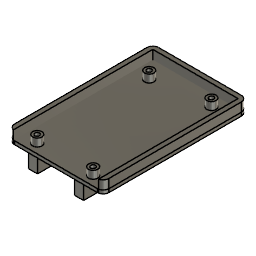
arduinoMount4080 (Autodesk Fusion 360 design; units mm, degrees)
part number: 2026-01-29-15-29-34-594
Autodesk Fusion 360 part; units mm, degrees
sketch "Sketch5" plane through (0, 0, 0) normal (0, 0, 1) x (1, 0, 0)
  line L0 (-41, -62.5) -> (41, -62.5)
  line L1 (41, -62.5) -> (41, 62.5)
  line L2 (41, 62.5) -> (-41, 62.5)
  line L3 (-41, 62.5) -> (-41, -62.5)
  line L4 (-41, -62.5) -> (41, 62.5) construction
  line L5 (41, -62.5) -> (-41, 62.5) construction
  line L6 (-37, 62.5) -> (-37, -62.5)
  line L7 (0, 62.5) -> (0, -62.5) construction
  line L8 (37, 62.5) -> (37, -62.5)
  line L9 (-10, -62.5) -> (10, -62.5) construction
  line L10 (23.95, -62.5) -> (16.05, -62.5)
  line L11 (16.05, -62.5) -> (16.05, 62.5)
  line L12 (16.05, 62.5) -> (23.95, 62.5)
  line L13 (23.95, 62.5) -> (23.95, -62.5)
  line L14 (-23.95, 62.5) -> (-23.95, -62.5)
  line L15 (-16.05, -62.5) -> (-16.05, 62.5)
  line L16 (-20, -62.5) -> (-20, 62.5) construction
  line L17 (20, -62.5) -> (20, 62.5) construction
  line L18 (-41, -58.5) -> (41, -58.5)
  line L19 (-23.95, -52.5) -> (-16.05, -52.5)
  line L20 (23.95, -52.5) -> (16.05, -52.5)
  line L21 (-27, -62.5) -> (-13, -62.5)
  line L22 (-13, -62.5) -> (-13, -72.5)
  line L23 (-13, -72.5) -> (-27, -72.5)
  line L24 (-27, -72.5) -> (-27, -62.5)
  line L25 (-27, -62.5) -> (-13, -72.5) construction
  line L26 (-27, -72.5) -> (-13, -62.5) construction
  circle A0 centre (-20, -67.5) radius 2.25
  line L27 (13, -72.5) -> (27, -72.5)
  line L28 (13, -62.5) -> (13, -72.5)
  line L29 (27, -72.5) -> (27, -62.5)
  circle A1 centre (20, -67.5) radius 2.25
  circle A2 centre (-24.25, -54.5) radius 4
  circle A3 centre (-24.25, -54.5) radius 2
  circle A4 centre (-23.75, 42.2) radius 4
  circle A5 centre (-23.75, 42.2) radius 2
  circle A6 centre (24.25, -54.5) radius 4
  circle A7 centre (24.25, -54.5) radius 2
  circle A8 centre (23.95, 48.5) radius 4
  circle A9 centre (23.95, 48.5) radius 2
  line L30 (-23.75, 42.2) -> (-23.75, 37.2315) construction
  line L31 (24.25, -54.5) -> (24.25, -58.0127) construction
  line L32 (-24.25, -54.5) -> (-24.25, -59.6718) construction
  line L33 (-41, 58.5) -> (41, 58.5)
  line L34 (-25.25, -56.2321) -> (-24.25, -56.8094)
  line L35 (-25.25, -56.2321) -> (-22.1514, -56.2321) construction
  line L36 (-23.25, -56.2321) -> (-24.25, -56.8094)
  line L37 (23.25, -56.2321) -> (24.25, -56.8094)
  line L38 (23.25, -56.2321) -> (25.465, -56.2321) construction
  line L39 (25.25, -56.2321) -> (24.25, -56.8094)
  line L40 (22.95, 46.7679) -> (23.95, 46.1906)
  line L41 (22.95, 46.7679) -> (25.5493, 46.7679) construction
  line L42 (24.95, 46.7679) -> (23.95, 46.1906)
  line L43 (-24.75, 40.4679) -> (-23.75, 39.8906)
  line L44 (-24.75, 40.4679) -> (-23.0984, 40.4679) construction
  line L45 (-22.75, 40.4679) -> (-23.75, 39.8906)
  dimension "d29" = 125
  dimension "d30" = 4
  dimension "d55" = 7.9
  dimension "d64" = 3.95
  dimension "d65" = 3.95
  dimension "d93" = 74
  dimension "d94" = 4
  dimension "d99" = 40
  dimension "d101" = 4
  dimension "d102" = 10
  dimension "d103" = 14
  dimension "d104" = 10
  dimension "d105" = 4.5
  dimension "d116" = 8
  dimension "d117" = 4
  dimension "d118" = 8
  dimension "d119" = 4
  dimension "d120" = 8
  dimension "d121" = 4
  dimension "d122" = 8
  dimension "d123" = 4
  dimension "d124" = 48.5
  dimension "d127" = 24.25
  dimension "d128" = 4
  dimension "d129" = 96.7
  dimension "d132" = 103
  dimension "d135" = 0.3
  dimension "d136" = 0.5
  dimension "d147" = 4
  dimension "d150" = 121
  dimension "d151" = 82
  dimension "d152" = 21
  dimension "d153" = 21
  dimension "d156" = 30
  dimension "d157" = 30
  dimension "d158" = 30
  dimension "d159" = 30
  constraint horizontal L0
  constraint perpendicular L0 L1
  constraint parallel L0 L2
  constraint parallel L1 L3
  constraint coincident L4 origin
  constraint coincident L5 origin
  constraint coincident L2 L6.start
  constraint coincident L0 L6.end
  constraint perpendicular L0 L6
  constraint midpoint L2 L7.start
  constraint midpoint L0 L7.end
  constraint symmetric L6.start L7 L8.start
  constraint symmetric L6.end L7 L8.end
  constraint horizontal L9
  constraint coincident L0 L9.start
  constraint horizontal L10
  constraint vertical L11
  constraint horizontal L12
  constraint vertical L13
  constraint coincident L0 L10.start
  constraint symmetric L7 L10.start L14.end
  constraint symmetric L7 L10.end L15.start
  constraint symmetric L7 L11.end L15.end
  constraint symmetric L7 L12.end L14.start
  constraint coincident L0 L16.start
  constraint coincident L2 L16.end
  constraint perpendicular L2 L16
  constraint symmetric L7 L16.start L17.start
  constraint symmetric L7 L16.end L17.end
  constraint coincident L2 L15.end
  constraint coincident L3 L18.start
  constraint coincident L1 L18.end
  constraint perpendicular L1 L18
  constraint coincident L14 L19.start
  constraint coincident L15 L19.end
  constraint perpendicular L15 L19
  constraint symmetric L7 L19.start L20.start
  constraint symmetric L7 L19.end L20.end
  constraint horizontal L21
  constraint vertical L22
  constraint horizontal L23
  constraint vertical L24
  constraint coincident L0 L21.start
  constraint midpoint L16.start L21
  constraint midpoint L25 A0.centre
  constraint symmetric L7 L21.start L29.end
  constraint symmetric L7 L21.end L28.start
  constraint symmetric L7 L22.end L27.start
  constraint symmetric L7 L23.end L27.end
  constraint symmetric L7 A0 A1
  constraint concentric A2 A3
  constraint concentric A4 A5
  constraint concentric A6 A7
  constraint concentric A8 A9
  constraint horizontal A2.centre A6.centre
  constraint vertical L30
  constraint coincident A4.centre A5.centre
  constraint vertical L31
  constraint coincident A6.centre A7.centre
  constraint vertical L32
  constraint coincident A2.centre A3.centre
  constraint coincident L3 L33.start
  constraint coincident L1 L33.end
  constraint perpendicular L1 L33
  constraint horizontal L35
  constraint coincident A3 L34.start
  constraint tangent A3 L34
  constraint coincident L32 L34.end
  constraint symmetric L32 L34.start L36.start
  constraint symmetric L32 L34.end L36.end
  constraint horizontal L38
  constraint coincident A7 L37.start
  constraint tangent A7 L37
  constraint coincident L31 L37.end
  constraint symmetric L31 L37.start L39.start
  constraint symmetric L31 L37.end L39.end
  constraint horizontal L41
  constraint coincident A9 L40.start
  constraint tangent A9 L40
  constraint coincident L13 L40.end
  constraint symmetric L13 L40.start L42.start
  constraint symmetric L13 L40.end L42.end
  constraint horizontal L44
  constraint coincident A5 L43.start
  constraint tangent A5 L43
  constraint coincident L30 L43.end
  constraint symmetric L30 L43.start L45.start
  constraint symmetric L30 L43.end L45.end
  measures "d29" distance of L0.end L1.end
  measures "d30" distance of L3 L6
  measures "d55" distance of L10.start L10.end
  measures "d64" distance of L14 L16
  measures "d65" distance of L15 L16
  measures "d93" distance of L6 L8
  measures "d94" distance of L1 L8
  measures "d99" distance of L16 L17
  measures "d101" distance of L0 L18
  measures "d102" distance of L16.start L19
  measures "d103" distance of L21.start L21.end
  measures "d104" distance of L21.start L23.end
  measures "d105" diameter of A0
  measures "d116" diameter of A2
  measures "d117" diameter of A3
  measures "d118" diameter of A4
  measures "d119" diameter of A5
  measures "d120" diameter of A6
  measures "d121" diameter of A7
  measures "d122" diameter of A8
  measures "d123" diameter of A9
  measures "d124" horizontal distance of A2.centre A6.centre
  measures "d127" distance of L7 A6.centre
  measures "d128" distance of L18 A6.centre
  measures "d129" vertical distance of A2.centre A4.centre
  measures "d132" vertical distance of A6.centre A8.centre
  measures "d135" horizontal distance of A6.centre A8.centre
  measures "d136" horizontal distance of A2.centre A4.centre
  measures "d147" distance of L2 L33
  measures "d150" distance of L0 L33
  measures "d151" distance of L1 L3
  measures "d152" distance of L3 L16
  measures "d153" distance of L1 L17
  measures "d156" angle of L34 L35
  measures "d157" angle of L37 L38
  measures "d158" angle of L40 L41
  measures "d159" angle of L43 L44
sketch "Sketch6" plane through (0, 0, 0) normal (0, 1, 0) x (1, 0, 0)
  line L0 (0, -56.6756) -> (0, 40) construction
  line L1 (-20, 40) -> (-20, 0) construction
  line L2 (20, 40) -> (20, 0) construction
  line L3 (20, 40) -> (20, 0) construction
  point P0 (0, -10.7)
  point P1 (0, -9.7)
  point P2 (0, -56.6756)
  point P3 (0, 40)
  point P4 (-20, 16)
  point P5 (20, 16)
  point P6 (-20, 12)
  point P7 (-20, 5)
  point P8 (20, 16)
  point P9 (20, 5)
  point P10 (-20, 24)
  point P11 (20, 24)
  point P12 (-24.75, 0)
  point P13 (-37, 0)
  point P14 (20, 24)
  point P15 (20, 12)
  point P16 (37, 0)
  point P17 (20, 16)
  point P18 (24.75, 0)
  point P19 (20, 5)
  point P20 (0, -3)
  dimension "d36" = 40
  dimension "d45" = 20
  dimension "d46" = 20
  dimension "d48" = 40
  dimension "d49" = 12
  dimension "d50" = 5
  dimension "d51" = 16
  dimension "d52" = 8
  dimension "d53" = 16
  dimension "d54" = 12.25
  dimension "d100" = 1
  dimension "d154" = 3
  dimension "d155" = 6.7
  constraint vertical P0 P1
  constraint vertical P1 origin
  constraint coincident P2 L0.start
  constraint coincident P3 L0.end
  constraint vertical L0
  constraint horizontal P4 P17
  constraint horizontal P3 L1.start
  constraint vertical P4 L1.start
  constraint coincident L1 P6
  constraint coincident L1 P7
  constraint symmetric P4 L0 P17
  constraint symmetric L0 L1.start L2.start
  constraint symmetric L0 L1.end L2.end
  constraint symmetric L0 P7 P19
  constraint coincident L1 P10
  constraint symmetric L0 P10 P14
  constraint symmetric L0 P6 P15
  constraint symmetric L0 P12 P18
  constraint symmetric L0 P13 P16
  constraint coincident L0 P20
  measures "d36" distance of P3 origin
  measures "d45" distance of P4 L0
  measures "d46" distance of P17 L0
  measures "d48" distance of L1.start L1.end
  measures "d49" distance of L1.end P6
  measures "d50" distance of L1.end P7
  measures "d51" distance of P4 L1.end
  measures "d52" distance of P4 P10
  measures "d53" distance of L1.start P10
  measures "d54" distance of P12 P13
  measures "d100" distance of P0 P1
  measures "d154" distance of origin P20
  measures "d155" distance of P1 P20
extrude "Extrude10" add sketch "Sketch5" along normal up to surface (3 mm away) contours L0 L3 L6 L18 | L0 L6 L14 L18 L21 | L3 L6 L18 L33 | L6 L14 L18 A2 A4 L33 | L2 L3 L6 L33 | L0 L14 L15 L18 L21 | L2 L6 L14 L33 | L14 L18 A2 | L14 A2 A3 L34 L36 | L0 L11 L15 L18 L21 | L14 L15 L18 L19 A2 | L14 L15 L19 A2 A4 L33 | L2 L14 L15 L33 | L14 L19 A2 | L14 L19 A2 A3 L36 | L11 L15 L18 L33 | L14 A4 A5 L43 L45 | L14 A4 A5 L43 | L2 L11 L15 L33 | L14 A3 L34 L36 | L14 A3 L36 | L0 L10 L11 L13 L18 | L11 L13 L18 L20 A6 | L14 A5 | L14 A5 | L11 L13 L20 A6 A8 L33 | L2 L11 L12 L13 L33 | L14 A5 L43 | L14 A5 L43 L45 | L14 A3 | L14 A3 | L0 L8 L13 L18 | L13 L18 A6 | L8 L13 L18 A6 A8 L33 | L2 L8 L13 L33 | L13 L20 A6 | L13 L20 A6 A7 L37 | L13 A6 A7 L37 L39 | L13 A8 A9 L42 | L13 A8 A9 L40 | L1 L8 L18 L33 | L1 L2 L8 L33 | L13 A7 L37 | L13 A7 L37 L39 | L0 L1 L8 L18 | L13 A9 | L13 A9 | L13 A7 | L13 A7 | L13 A9 L42 | L13 A9 L40 makes body 1
extrude "Extrude21" add sketch "Sketch5" along normal up to surface (6.7 mm away) from surface at 3 separate body contours L14 A2 A3 L34 L36 | L14 L19 A2 | L14 L19 A2 A3 L36 | L14 A4 A5 L43 L45 | L14 A4 A5 L43 | L13 L20 A6 | L13 L20 A6 A7 L37 | L13 A6 A7 L37 L39 | L13 A8 A9 L42 | L13 A8 A9 L40 makes body 2 at (27.9301, 48.8983, 7.4667) makes body 3 at (-19.7699, 41.8017, 5.2333) makes body 4 at (28.2301, -54.1017, 7.4667) makes body 5 at (-20.2699, -54.8983, 5.2333)
extrude "Extrude14" add sketch "Sketch5" against normal up to surface (12 mm away) separate body contours L0 L14 L15 L18 L21 | L14 L15 L18 L19 A2 | L14 L15 L19 A2 A4 L33 | L2 L14 L15 L33 | L14 L19 A2 | L14 L19 A2 A3 L36 | L14 A4 A5 L43 L45 | L14 A3 L36 | L0 L10 L11 L13 L18 | L11 L13 L18 L20 A6 | L14 A5 | L11 L13 L20 A6 A8 L33 | L14 A5 L43 L45 | L14 A3 | L13 L20 A6 | L13 L20 A6 A7 L37 | L13 A8 A9 L40 | L13 A7 L37 | L13 A9 | L13 A7 | L13 A9 L40 picked at (-23.3174, 42.5524) picked at (-23.3833, -54.5) picked at (23.2836, 48.4806) picked at (23.4056, -54.3292) makes body 6 at (-23.95, 20.8333, -4) makes body 7 at (23.95, 18.1667, -4)
sketch "Sketch8" plane through (-16.05, 0, 0) normal (1, 0, 0) x (0, 1, 0)
  line L0 (-62.5, -12) -> (62.5, -12)
  line L1 (62.5, -12) -> (62.5, 0)
  line L2 (-62.5, -5) -> (62.5, -5)
  line L3 (62.5, -5) -> (-62.5, -5)
  line L4 (62.5, 0) -> (-62.5, 0)
  line L5 (-62.5, 0) -> (-62.5, -12)
  point P0 (-62.5, 0)
  dimension "d59" = 5
  constraint coincident L1 L2.end
  constraint perpendicular L1 L2
  constraint coincident L2.start L5
  measures "d59" distance of L2.start P0
extrude "Extrude15" [suppressed]
fillet "Fillet1" [suppressed]
sketch "Sketch9" plane through (-23.95, 0, 0) normal (-1, 0, 0) x (0, -1, 0)
  line L0 (-62.5, -12) -> (62.5, -12)
  line L1 (-62.5, 0) -> (-62.5, -12)
  line L2 (-62.5, -5) -> (62.5, -5)
  line L3 (-62.5, 0) -> (62.5, 0)
  line L4 (62.5, 0) -> (-62.5, 0)
  line L5 (62.5, -12) -> (62.5, 0)
  dimension "d67" = 5
  constraint coincident L1 L2.start
  constraint coincident L2.end L5
  measures "d67" distance of L2 L3
extrude "Extrude16" [suppressed]
fillet "Fillet2" [suppressed]
mirror "Mirror1" [suppressed]
extrude "Extrude18" [suppressed]
pipe "Pipe1" [suppressed]
extrude "Extrude19" [suppressed]
pipe "Pipe2" [suppressed]
extrude "Extrude20" add sketch "Sketch5" along normal up to surface (10.7 mm away) separate body contours L0 L3 L6 L18 | L3 L6 L18 L33 | L2 L3 L6 L33 | L2 L6 L14 L33 | L2 L14 L15 L33 | L2 L11 L15 L33 | L2 L11 L12 L13 L33 | L2 L8 L13 L33 | L1 L8 L18 L33 | L1 L2 L8 L33 | L0 L1 L8 L18 makes body 8
fillet "Fillet4" [suppressed]
fillet "Fillet5" [suppressed]
fillet "Fillet7" radius 5 4 edges at (41, -62.5, 1.5) (-41, -62.5, 1.5) (-41, 62.5, 1.5) (41, 62.5, 1.5) on bodies 1 8
fillet "Fillet7" radius 5 4 edges at (41, -62.5, 5.35) (-41, -62.5, 5.35) (-41, 62.5, 5.35) (41, 62.5, 5.35) on bodies 1 8
equation "d46 = d45"
equation "d47 = 8 mm"
equation "d51 = d48 / 2 - d47 / 2"
equation "d59 = d50"
equation "d67 = d50"
equation "d101 = d30"
equation "d116 = d118"
equation "d118 = d117 + 4 mm"
equation "d120 = d118"
equation "d122 = d118"
equation "d127 = d124 / 2"
equation "d147 = d30"
